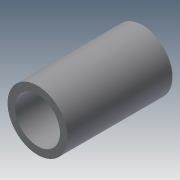
# Autodesk Inventor part: servoGear
Saved by Autodesk Inventor 2018 (Build 220112000, 112)
## iProperties
Created: 2020-02-25
Part Number: servoGear
Material: Generic
Document SubType Name: Modeling
Designer: anirudh
Density: 1 g/cm^3
Appearance: Default
Author: anirudh
Autodesk Inventor part; units mm, degrees
ref_plane "YZ Plane" through (0, 0, 0) normal (1, 0, 0) x (0, 1, 0)
ref_plane "XZ Plane" through (0, 0, 0) normal (0, 1, 0) x (-1, 0, 0)
ref_plane "XY Plane" through (0, 0, 0) normal (0, 0, 1) x (1, 0, 0)
sketch "Sketch1" plane through (0, 0, 0) normal (0, 0, 1) x (1, 0, 0)
  circle A0 centre (0, 0) radius 2.3813
  circle A1 centre (0, 0) radius 4.7625
  dimension "d1" = 4.7625
  constraints: 2 centre point, 1 coincident
  measures "d1" diameter of A0
extrude "Extrusion2" add sketch "Sketch1" along normal blind 11.1125
body "Solid2"
